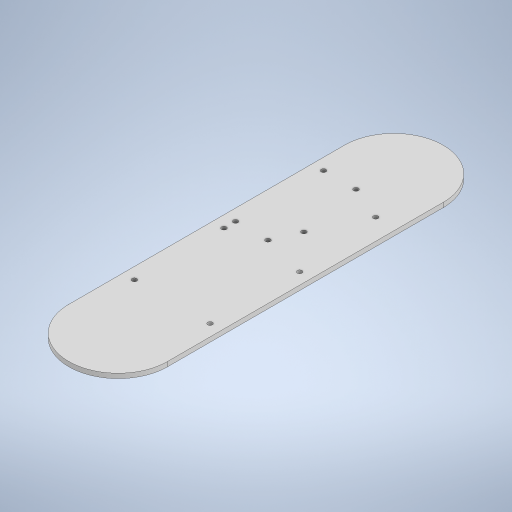
# Autodesk Inventor part: electronics_layout_v1
Saved by Autodesk Inventor 2023.1 (Build 271208000, 208)
## iProperties
Created: 2026-05-19
Part Number: electronics_layout_v1
Material: Generic
Document SubType Name: Modeling
Designer: Lars
Density: 1 g/cm^3
Appearance: Default
Author: Lars
Autodesk Inventor part; units mm, degrees
ref_plane "YZ Plane" through (0, 0, 0) normal (1, 0, 0) x (0, 1, 0)
ref_plane "XZ Plane" through (0, 0, 0) normal (0, 1, 0) x (-1, 0, 0)
ref_plane "XY Plane" through (0, 0, 0) normal (0, 0, 1) x (1, 0, 0)
sketch "Sketch1" plane through (0, 0, 0) normal (0, 1, 0) x (-1, 0, 0)
  line L0 (0, 0) -> (49, 0) construction
  line L1 (49, 0) -> (49, -58) construction
  line L2 (49, -58) -> (0, -58) construction
  line L3 (0, -58) -> (0, 0) construction
  line L4 (53.5, 32) -> (-4.5, 32) construction
  line L5 (-4.5, 32) -> (-4.5, -62) construction
  line L6 (-4.5, -62) -> (53.5, -62) construction
  line L7 (53.5, -62) -> (53.5, 32) construction
  line L8 (53.5, -58) -> (-4.5, -58) construction
  line L9 (24.5, -62) -> (24.5, -133) construction
  line L10 (49, -65.5) -> (28, -65.5) construction
  line L11 (28, -65.5) -> (28, -122.5) construction
  line L12 (28, -122.5) -> (49, -122.5) construction
  line L13 (49, -122.5) -> (49, -65.5) construction
  line L14 (24.5, -94) -> (28, -94) construction
  line L15 (45.5, -122.5) -> (31.5, -122.5) construction
  line L16 (31.5, -122.5) -> (31.5, -140.5) construction
  line L17 (31.5, -140.5) -> (45.5, -140.5) construction
  line L18 (45.5, -140.5) -> (45.5, -122.5) construction
  line L19 (21, -81.75) -> (6, -81.75) construction
  line L20 (6, -81.75) -> (6, -113.25) construction
  line L21 (6, -113.25) -> (21, -113.25) construction
  line L22 (21, -113.25) -> (21, -81.75) construction
  line L23 (24.5, -97.5) -> (21, -97.5) construction
  circle A0 centre (49, -122.5) radius 1.5
  circle A1 centre (49, -65.5) radius 1.5
  circle A2 centre (28, -65.5) radius 1.5
  circle A3 centre (28, -122.5) radius 1.5
  circle A4 centre (49, -58) radius 1.5
  circle A5 centre (0, -58) radius 1.5
  circle A6 centre (0, 0) radius 1.5
  circle A7 centre (49, 0) radius 1.5
  circle A8 centre (21, -81.75) radius 1.5
  circle A9 centre (6, -113.25) radius 1.5
  line L24 (53.5, 32) -> (-4.5, 32) construction
  line L25 (-4.5, 32) -> (-4.5, -140.5) construction
  line L26 (-4.5, -140.5) -> (53.5, -140.5) construction
  line L27 (53.5, -140.5) -> (53.5, 32) construction
  line L28 (56.5, 35) -> (-7.5, 35) construction
  line L29 (-7.5, 35) -> (-7.5, -143.5)
  line L30 (-7.5, -143.5) -> (56.5, -143.5) construction
  line L31 (56.5, -143.5) -> (56.5, 35)
  arc A10 (56.5, 35) -> (-7.5, 35) centre (24.5, 35) ccw
  arc A11 (-7.5, -143.5) -> (56.5, -143.5) centre (24.5, -143.5) ccw
  point P0 (24.5, -58)
  point P1 (38.5, -122.5)
  point P2 (38.5, -140.5)
  point P3 (53.5, -15)
  point P4 (-4.5, -15)
  point P5 (24.5, 32)
  dimension "d0" = 49
  dimension "d1" = 58
  dimension "d2" = 58
  dimension "d3" = 94
  dimension "d4" = 4
  dimension "d7" = 71
  dimension "d8" = 21
  dimension "d9" = 57
  dimension "d10" = 32
  dimension "d11" = 3.5
  dimension "d12" = 14
  dimension "d13" = 18
  dimension "d14" = 15
  dimension "d15" = 31.5
  dimension "d16" = 3.5
  dimension "d17" = 3
  dimension "d18" = 3
  dimension "d19" = 3
  dimension "d20" = 3
  dimension "d21" = 3
  dimension "d22" = 3
  dimension "d23" = 3
  dimension "d24" = 3
  dimension "d25" = 3
  dimension "d26" = 3
  dimension "d27" = 3
  constraints: 64 end point, 14 parallel, 13 midpoint, 12 centre point, 10 coincident, 8 perpendicular, 8 point on line, 7 horizontal, 4 point on circle, 4 tangent, 1 vertical, 3 other
  measures "d0" distance of L1.end L2.end
  measures "d1" distance of L0.end L1.end
  measures "d2" distance of L5.end L6.end
  measures "d3" distance of L6.end L4.start
  measures "d4" distance between parallel lines of L6 L2
  measures "d7" distance of L9.start L9.end
  measures "d8" distance of L12.end L11.end
  measures "d9" distance of L11.end L10.end
  measures "d10" distance between parallel lines of L6 L14
  measures "d11" distance of L14.start L14.end
  measures "d12" distance of L17.end L16.end
  measures "d13" distance of L16.end L15.end
  measures "d14" distance of L21.end L20.end
  measures "d15" distance of L20.end L19.end
  measures "d16" distance of L23.end L23.start
  measures "d17" diameter of A0
  measures "d18" diameter of A1
  measures "d19" diameter of A2
  measures "d20" diameter of A3
  measures "d21" diameter of A4
  measures "d22" diameter of A5
  measures "d23" diameter of A6
  measures "d24" diameter of A7
  measures "d25" diameter of A8
  measures "d26" diameter of A9
  measures "d27" distance between parallel lines of L27 L31
extrude "Extrusion1" add sketch "Sketch1" along normal blind 3
body "Solid1"
